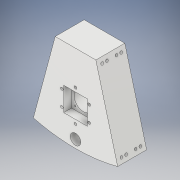
# Autodesk Inventor part: CA001
Saved by Autodesk Inventor 2017 SP1 (Build 210196100, 196)
## iProperties
Created: 2017-06-04
Part Number: CA001
Material: ABS Plastic
Document SubType Name: Modeling
Designer: Zach
Density: 1.06 g/cm^3
Appearance: CR White
Author: Zach
Autodesk Inventor part; units mm, degrees
ref_plane "YZ Plane" through (0, 0, 0) normal (1, 0, 0) x (0, 1, 0)
ref_plane "XZ Plane" through (0, 0, 0) normal (0, 1, 0) x (-1, 0, 0)
ref_plane "XY Plane" through (0, 0, 0) normal (0, 0, 1) x (1, 0, 0)
sketch "Sketch1" plane through (0, 0, 0) normal (0, 0, 1) x (1, 0, 0)
  line L0 (0, 0) -> (160, 0)
  line L1 (160, 0) -> (118.589, 154.5481)
  line L2 (41.411, 154.5481) -> (0, 0)
  line L3 (41.411, 154.5481) -> (118.589, 154.5481)
  dimension "d0" = 160
  dimension "d1" = 160
  dimension "d2" = 75
  dimension "d8" = 75
  constraints: 8 end point, 2 horizontal
  measures "d0" distance of L0.start L0.end
  measures "d1" distance of L1.end L0.end
  measures "d2" angle of L1 L0
  measures "d8" angle of L0 L2
extrude "Extrusion1" add sketch "Sketch1" along normal blind 55
sketch "Sketch7" plane through (0, 0, 0) normal (0, 0, -1) x (-1, 0, 0)
  circle A0 centre (-80, 304.672) radius 315 construction
  line L0 (0, 0) -> (-160, 0) projected
  arc A1 (-160, 0) -> (0, 0) centre (-80, 304.672) ccw
  dimension "d28" = 630
  constraints: 4 point on circle, 2 centre point, 1 concentric
  measures "d28" diameter of A0
extrude "Extrusion6" add sketch "Sketch7" against normal blind 55
sketch "Sketch19" plane through (0, 0, 0) normal (0, 0, -1) x (-1, 0, 0)
  circle A0 centre (-80, 60) radius 55
  line L0 (-118.589, 154.5481) -> (-41.411, 154.5481) projected
  point P0 (0, 0)
  point P1 (-80, 154.5481)
  dimension "d112" = 110
  dimension "d113" = 60
  constraints: 1 centre point, 1 midpoint, 1 vertical alignment
  measures "d112" diameter of A0
  measures "d113" vertical distance of point (0, 0) A0.centre
extrude "Extrusion19" cut sketch "Sketch19" against normal blind 13
sketch "Sketch20" plane through (80, 60, 13) normal (0, 0, -1) x (-1, 0, 0)
  circle A0 centre (0, 0) radius 55 construction
  circle A1 centre (0, 0) radius 17.5
  point P0 (80, -60)
  dimension "d116" = 35
  constraints: 1 centre point, 1 coincident
  measures "d116" diameter of A1
extrude "Extrusion20" cut sketch "Sketch20" against normal through all
sketch "Sketch21" plane through (0, 0, 55) normal (0, 0, 1) x (1, 0, 0)
  circle A0 centre (80, 60) radius 17.5 construction
  line L0 (57.5, 37.5) -> (102.5, 37.5)
  line L1 (102.5, 37.5) -> (102.5, 82.5)
  line L2 (102.5, 82.5) -> (57.5, 82.5)
  line L3 (57.5, 82.5) -> (57.5, 37.5)
  point P0 (0, 0)
  point P1 (57.5, 60)
  point P2 (80, 82.5)
  dimension "d119" = 45
  dimension "d120" = 45
  constraints: 8 end point, 2 midpoint, 2 parallel, 1 centre point, 1 horizontal, 1 horizontal alignment, 1 perpendicular, 1 vertical alignment
  measures "d119" distance of L2.end L1.end
  measures "d120" distance of L1.end L0.end
extrude "Extrusion21" cut sketch "Sketch21" against normal blind 15
sketch "Sketch23" plane through (0, 0, 40) normal (0, 0, 1) x (1, 0, 0)
  line L0 (64.5, 75.5) -> (95.5, 75.5) construction
  line L1 (95.5, 75.5) -> (95.5, 44.5) construction
  line L2 (95.5, 44.5) -> (64.5, 44.5) construction
  line L3 (64.5, 44.5) -> (64.5, 75.5) construction
  circle A0 centre (80, 60) radius 17.5 construction
  circle A1 centre (95.5, 75.5) radius 1.5
  circle A2 centre (95.5, 44.5) radius 1.5
  circle A3 centre (64.5, 44.5) radius 1.5
  circle A4 centre (64.5, 75.5) radius 1.5
  point P0 (0, 0)
  point P1 (64.5, 60)
  point P2 (80, 75.5)
  dimension "d126" = 31
  dimension "d127" = 31
  dimension "d128" = 3
  dimension "d129" = 3
  dimension "d130" = 3
  dimension "d131" = 3
  constraints: 8 end point, 5 centre point, 4 coincident, 2 midpoint, 2 parallel, 1 horizontal, 1 horizontal alignment, 1 perpendicular, 1 vertical alignment
  measures "d126" distance of L1.end L2.end
  measures "d127" distance of L0.end L1.end
  measures "d128" diameter of A1
  measures "d129" diameter of A2
  measures "d130" diameter of A3
  measures "d131" diameter of A4
extrude "Extrusion23" cut sketch "Sketch23" against normal through all
sketch "Sketch25" plane through (80, 60, 13) normal (0, 0, -1) x (-1, 0, 0)
  circle A0 centre (0, 30) radius 2.5
  circle A1 centre (0, 0) radius 55 construction
  circle A2 centre (-25.9808, 15) radius 2.5
  circle A3 centre (-25.9808, -15) radius 2.5
  circle A4 centre (0, -30) radius 2.5
  circle A5 centre (25.9808, -15) radius 2.5
  circle A6 centre (25.9808, 15) radius 2.5
  point P0 (80, -60)
  dimension "d138" = 5
  dimension "d139" = 30
  dimension "d142" = 360
  constraints: 6 centre point, 1 vertical alignment, 13 other
  measures "d138" diameter of A0
  measures "d139" distance of A0.centre A1.centre
extrude "Extrusion25" cut sketch "Sketch25" against normal through all
sketch "Sketch26" plane through (80, 60, 13) normal (0, 0, -1) x (-1, 0, 0)
  circle A0 centre (15.5, -15.5) radius 1.5 projected
  circle A1 centre (-15.5, -15.5) radius 1.5 projected
  circle A2 centre (-15.5, 15.5) radius 1.5 projected
  circle A3 centre (15.5, 15.5) radius 1.5 projected
  circle A4 centre (15.5, -15.5) radius 3.5
  circle A5 centre (-15.5, -15.5) radius 1.5 projected
  circle A6 centre (-15.5, -15.5) radius 3.5
  circle A7 centre (-15.5, 15.5) radius 3.5
  circle A8 centre (15.5, 15.5) radius 3.5
  point P0 (80, -60)
  dimension "d146" = 7
  dimension "d147" = 7
  dimension "d148" = 7
  dimension "d149" = 7
  constraints: 4 centre point, 4 coincident
  measures "d146" diameter of A4
  measures "d147" diameter of A6
  measures "d148" diameter of A7
  measures "d149" diameter of A8
extrude "Extrusion26" cut sketch "Sketch26" against normal blind 20 contours A0 | A1 | A2 | A3 | A4 | A6 | A7 | A8
sketch "Sketch27" plane through (0, 0, 55) normal (0, 0, 1) x (1, 0, 0)
  circle A0 centre (80, 4.836) radius 10
  line L0 (118.589, 154.5481) -> (41.411, 154.5481) construction
  line L1 (80, 154.5481) -> (80, -10.328) construction
  arc A1 (0, 0) -> (160, 0) centre (80, 304.672) ccw construction
  dimension "d152" = 20
  dimension "d153" = 15.164
  constraints: 2 end point, 1 centre point, 1 midpoint, 1 perpendicular, 1 point on circle, 1 point on line
  measures "d152" diameter of A0
  measures "d153" distance of L1.end A0.centre
extrude "Extrusion27" cut sketch "Sketch27" against normal through all
sketch "Sketch28" plane through (41.411, 154.5481, 0) normal (-0.9659, 0.2588, 0) x (0, 0, 1)
  line L0 (9.525, -150.46) -> (9.525, -9.54) construction
  circle A0 centre (9.525, -150.46) radius 2.5
  circle A1 centre (9.525, -9.54) radius 2.5
  line L1 (0, 0) -> (0, -160) projected
  circle A2 centre (18.4199, -9.54) radius 2.5
  circle A3 centre (36.5801, -9.54) radius 2.5
  circle A4 centre (45.475, -9.54) radius 2.5
  line L2 (55, 0) -> (55, -160) projected
  circle A5 centre (18.4199, -150.46) radius 2.5
  circle A6 centre (36.5801, -150.46) radius 2.5
  circle A7 centre (45.475, -150.46) radius 2.5
  point P0 (9.525, -80)
  point P1 (0, -80)
  dimension "d156" = 140.92
  dimension "d157" = 5
  dimension "d158" = 5
  dimension "d159" = 9.525
  dimension "d160" = 5
  dimension "d161" = 5
  dimension "d162" = 5
  dimension "d163" = 18.4199
  dimension "d164" = 18.4199
  dimension "d165" = 9.525
  dimension "d166" = 5
  dimension "d167" = 5
  dimension "d168" = 5
  constraints: 8 centre point, 7 horizontal alignment, 3 vertical alignment, 2 coincident, 2 end point, 2 midpoint, 1 vertical
  measures "d156" distance of L0.start L0.end
  measures "d157" diameter of A0
  measures "d158" diameter of A1
  measures "d159" distance from line of L1 L0.end
  measures "d160" diameter of A2
  measures "d161" diameter of A3
  measures "d162" diameter of A4
  measures "d163" distance from line of L1 A2.centre
  measures "d164" distance from line of L2 A3.centre
  measures "d165" distance from line of L2 A4.centre
  measures "d166" diameter of A5
  measures "d167" diameter of A6
  measures "d168" diameter of A7
extrude "Extrusion28" cut sketch "Sketch28" against normal blind 25
sketch "Sketch29" plane through (118.589, 154.5481, 55) normal (0.9659, 0.2588, 0) x (0, 0, -1)
  line L0 (9.525, -150.46) -> (9.525, -9.54) construction
  circle A0 centre (9.525, -150.46) radius 2.5
  circle A1 centre (9.525, -9.54) radius 2.5
  circle A2 centre (18.4199, -9.54) radius 2.5
  circle A3 centre (36.5801, -9.54) radius 2.5
  circle A4 centre (45.475, -9.54) radius 2.5
  circle A5 centre (18.4199, -150.46) radius 2.5
  circle A6 centre (36.5801, -150.46) radius 2.5
  circle A7 centre (45.475, -150.46) radius 2.5
  line L1 (0, -160) -> (0, 0) projected
  line L2 (55, -160) -> (55, 0) projected
  point P0 (9.525, -80)
  point P1 (0, -80)
  point P2 (0, -80)
  dimension "d169" = 140.92
  dimension "d170" = 5
  dimension "d171" = 5
  dimension "d173" = 5
  dimension "d174" = 5
  dimension "d175" = 5
  dimension "d179" = 5
  dimension "d180" = 5
  dimension "d181" = 5
  dimension "d184" = 9.525
  dimension "d185" = 18.4199
  dimension "d186" = 9.525
  dimension "d187" = 18.4199
  constraints: 8 centre point, 8 horizontal alignment, 3 vertical alignment, 2 coincident, 2 end point, 2 midpoint, 1 vertical
  measures "d169" distance of L0.start L0.end
  measures "d170" diameter of A0
  measures "d171" diameter of A1
  measures "d173" diameter of A2
  measures "d174" diameter of A3
  measures "d175" diameter of A4
  measures "d179" diameter of A5
  measures "d180" diameter of A6
  measures "d181" diameter of A7
  measures "d184" distance from line of L1 L0.start
  measures "d185" distance from line of L1 A5.centre
  measures "d186" distance from line of L2 A7.centre
  measures "d187" distance from line of L2 A6.centre
extrude "Extrusion29" cut sketch "Sketch29" against normal blind 25
body "Solid1"
